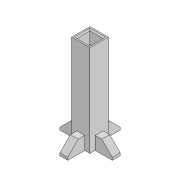
# Autodesk Inventor part: FlipperStand
Saved by Autodesk Inventor 2021 (Build 250183000, 183)
## iProperties
Created: 2021-04-02
Part Number: FlipperStand
Material: Generic
Document SubType Name: Modeling
Designer: Tran Duc Viet
Mass: 1881.33 g
Surface Area: 1496.44 cm^2
Volume: 1881.33 cm^3
Density: 1 g/cm^3
Appearance: Default
Author: Tran Duc Viet
Autodesk Inventor part; units mm, degrees
ref_plane "YZ Plane" through (0, 0, 0) normal (1, 0, 0) x (0, 1, 0)
ref_plane "XZ Plane" through (0, 0, 0) normal (0, 1, 0) x (-1, 0, 0)
ref_plane "XY Plane" through (0, 0, 0) normal (0, 0, 1) x (1, 0, 0)
sketch "Sketch1" plane through (0, 0, 0) normal (0, 1, 0) x (-1, 0, 0)
  line L0 (0, 0) -> (70, 0)
  line L1 (70, 0) -> (70, -70)
  line L2 (70, -70) -> (0, -70)
  line L3 (0, -70) -> (0, 0)
  dimension "d0" = 70
  dimension "d1" = 70
  constraints: 8 end point, 2 parallel, 1 horizontal, 1 perpendicular
  measures "d0" distance of L1.end L2.end
  measures "d1" distance of L0.end L1.end
extrude "Extrusion1" add sketch "Sketch1" along normal blind 350
sketch "Sketch2" plane through (0, 350, 0) normal (0, 1, 0) x (1, 0, 0)
  line L0 (-10, 10) -> (-60, 10)
  line L1 (-60, 10) -> (-60, 60)
  line L2 (-60, 60) -> (-10, 60)
  line L3 (-10, 60) -> (-10, 10)
  line L4 (-70, 0) -> (0, 0) projected
  line L5 (0, 0) -> (0, 70) projected
  dimension "d4" = 50
  dimension "d5" = 50
  dimension "d6" = 10
  dimension "d7" = 10
  constraints: 8 end point, 2 parallel, 1 horizontal, 1 perpendicular
  measures "d4" distance of L1.end L2.end
  measures "d5" distance of L0.end L1.end
  measures "d6" distance between parallel lines of L4 L0
  measures "d7" distance between parallel lines of L5 L3
extrude "Extrusion2" cut sketch "Sketch2" against normal blind 50
chamfer "Chamfer1" distance 5 angle 45 4 edges at (-60, 350, -35) (-35, 350, -60) (-10, 350, -35) (-35, 350, -10)
sketch "Sketch3" plane through (0, 0, 0) normal (0, -1, 0) x (1, 0, 0)
  line L0 (-20, 65) -> (-50, 65)
  line L1 (-50, 65) -> (-50, -135)
  line L2 (-50, -135) -> (-20, -135)
  line L3 (-20, -135) -> (-20, 65)
  line L4 (65, -20) -> (-135, -20)
  line L5 (-135, -20) -> (-135, -50)
  line L6 (-135, -50) -> (65, -50)
  line L7 (65, -50) -> (65, -20)
  line L8 (0, 0) -> (0, -70) projected
  line L9 (0, -70) -> (-70, -70) projected
  line L10 (-70, -70) -> (-70, 0) projected
  point P0 (-50, -50)
  point P1 (-20, -50)
  point P2 (-20, -20)
  point P3 (-50, -20)
  dimension "d14" = 200
  dimension "d15" = 200
  dimension "d16" = 20
  dimension "d17" = 30
  dimension "d18" = 30
  dimension "d19" = 20
  dimension "d20" = 65
  dimension "d21" = 65
  constraints: 16 end point, 4 parallel, 2 horizontal, 2 perpendicular
  measures "d14" distance of L0.end L1.end
  measures "d15" distance of L5.end L6.end
  measures "d16" distance between parallel lines of L8 L3
  measures "d17" distance of L1.end L2.end
  measures "d18" distance of L4.end L5.end
  measures "d19" distance between parallel lines of L9 L6
  measures "d20" distance between parallel lines of L9 L2
  measures "d21" distance between parallel lines of L10 L5
extrude "Extrusion3" add sketch "Sketch3" against normal blind 50 contours L3 L4 L1 L0 | L4 L8 L6 L3 | L3 L6 L1 L4 | L1 L6 L10 L4 | L3 L9 L1 L6 | L4 L7 L6 L8 | L10 L6 L5 L4 | L3 L2 L1 L9
chamfer "Chamfer2" distance 40 angle 45 4 edges at (-35, 50, 65) (-135, 50, -35) (-35, 50, -135) (65, 50, -35)
body "Solid1"
